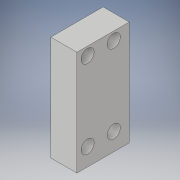
# Autodesk Inventor part: 8.2a
Saved by Autodesk Inventor 2017.3 (Build 213256000, 256)
## iProperties
Created: 2017-05-02
Part Number: 8.2a
Material: Generic
Document SubType Name: Modeling
Designer: rbibb
Density: 1 g/cm^3
Appearance: Default
Author: rbibb
Autodesk Inventor part; units mm, degrees
ref_plane "YZ Plane" through (0, 0, 0) normal (1, 0, 0) x (0, 1, 0)
ref_plane "XZ Plane" through (0, 0, 0) normal (0, 1, 0) x (-1, 0, 0)
ref_plane "XY Plane" through (0, 0, 0) normal (0, 0, 1) x (1, 0, 0)
sketch "Sketch1" plane through (0, 0, 0) normal (1, 0, 0) x (0, 1, 0)
  line L0 (14.9656, 6.7345) -> (-10.4344, 6.7345)
  line L1 (-10.4344, 6.7345) -> (-10.4344, -5.9655)
  line L2 (-10.4344, -5.9655) -> (14.9656, -5.9655)
  line L3 (14.9656, -5.9655) -> (14.9656, 6.7345)
  point P0 (0, 0)
  dimension "d0" = 25.4
  dimension "d1" = 12.7
  constraints: 8 end point, 2 parallel, 1 horizontal, 1 perpendicular
  measures "d0" distance of L1.end L2.end
  measures "d1" distance of L0.end L1.end
extrude "Extrusion1" add sketch "Sketch1" along normal blind 6.35
sketch "Sketch2" plane through (6.35, 0, 0) normal (1, 0, 0) x (0, 0, -1)
  circle A0 centre (-4.1568, 12.913) radius 1.5875
  line L0 (-6.7345, 14.9656) -> (-6.7345, -10.4344) projected
  line L1 (5.9655, 14.9656) -> (-6.7345, 14.9656) projected
  circle A1 centre (2.1932, 12.913) radius 1.5875
  circle A2 centre (-4.1568, -6.137) radius 1.5875
  circle A3 centre (2.1932, -6.137) radius 1.5875
  point P0 (0, 0)
  dimension "d4" = 3.175
  dimension "d9" = 6.35
  dimension "d12" = 19.05
  constraints: 4 centre point, 1 horizontal, 1 vertical, 6 other
  measures "d4" diameter of A0
  measures "d9" distance of A0.centre A1.centre
  measures "d12" distance of A0.centre A2.centre
extrude "Extrusion2" cut sketch "Sketch2" against normal blind 6.35
equation "\"d1\" = 0.5 * d0"
equation "\"d2\" = 0.5 * d1"
equation "\"d4\" = 0.5 * d2"
equation "\"d15\" = 0.5 * d1"
body "Solid1"
